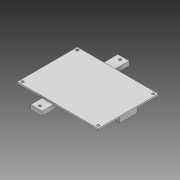
# Autodesk Inventor part: soporte_odroid_xu3
Saved by Autodesk Inventor 2018 (Build 220112000, 112)
## iProperties
Created: 2019-01-29
Part Number: soporte_odroid_xu3
Material: Genérico
Document SubType Name: Modeling
Designer: becar
Density: 1 g/cm^3
Appearance: Valor por defecto
Author: becar
Autodesk Inventor part; units mm, degrees
ref_plane "YZ Plane" through (0, 0, 0) normal (1, 0, 0) x (0, 1, 0)
ref_plane "XZ Plane" through (0, 0, 0) normal (0, 1, 0) x (-1, 0, 0)
ref_plane "XY Plane" through (0, 0, 0) normal (0, 0, 1) x (1, 0, 0)
sketch "Boceto1" plane through (0, 0, 0) normal (0, 0, 1) x (1, 0, 0)
  line L0 (0, 0) -> (87, 0)
  line L1 (87, 63) -> (0, 63)
  circle A0 centre (0, 63) radius 1.5
  circle A1 centre (87, 63) radius 1.5
  circle A2 centre (87, 0) radius 1.5
  circle A3 centre (0, 0) radius 1.5
  line L2 (0, -3) -> (87, -3)
  line L3 (87, -3) -> (90, -3)
  line L4 (90, -3) -> (90, 63)
  line L5 (90, 63) -> (90, 66)
  line L6 (90, 66) -> (0, 66)
  line L7 (0, 66) -> (-3, 66)
  line L8 (-3, 66) -> (-3, -3)
  line L9 (-3, -3) -> (0, -3)
  dimension "d0" = 87
  dimension "d1" = 63
  dimension "d2" = 3
  dimension "d3" = 3
  dimension "d4" = 3
  dimension "d5" = 3
  dimension "d8" = 3
  dimension "d9" = 3
  dimension "d10" = 3
  constraints: 20 end point, 4 centre point, 4 coincident, 4 point on line, 3 perpendicular, 2 horizontal, 1 collinear
  measures "d0" distance of L0.start L0.end
  measures "d1" distance of L0.end L1.start
  measures "d2" diameter of A0
  measures "d3" diameter of A1
  measures "d4" diameter of A2
  measures "d5" diameter of A3
  measures "d8" distance of L2.end L3.end
  measures "d9" distance of L4.end L5.end
  measures "d10" distance of L6.end L7.end
extrude "Extrusión1" add sketch "Boceto1" along normal blind 2
sketch "Boceto2" plane through (0, 0, 0) normal (0, 0, -1) x (-1, 0, 0)
  line L0 (0, 0) -> (0, -12)
  circle A0 centre (0, 63) radius 1.5 projected
  line L1 (0, 63) -> (0, 80)
  line L2 (0, 80) -> (-32, 80)
  line L3 (0, -12) -> (-32, -12)
  circle A1 centre (-32, 80) radius 1.5
  circle A2 centre (-32, -12) radius 1.5
  line L4 (-32, 80) -> (-25.5, 80)
  line L5 (-25.5, 80) -> (-25.5, 84)
  line L6 (-25.5, 84) -> (-38.5, 84)
  line L7 (-38.5, 84) -> (-38.5, 66)
  line L8 (-90, 66) -> (3, 66) projected
  line L9 (-25.5, 80) -> (-25.5, 66)
  line L10 (-38.5, -12) -> (-38.5, -2.9941)
  line L11 (-38.5, -12) -> (-38.5, -16)
  line L12 (-38.5, -16) -> (-25.5, -16)
  line L13 (-25.5, -16) -> (-25.5, -3)
  line L14 (3, -3) -> (-90, -3) projected
  line L15 (3, 66) -> (3, -3) projected
  line L16 (3, 31.5) -> (3, 41.5)
  line L17 (3, 31.5) -> (3, 21.5)
  line L18 (-90, -3) -> (-90, 66) projected
  line L19 (-90, 21.5) -> (-90, 41.5)
  line L20 (-90, 41.5) -> (-38.5, 41.5)
  line L21 (-38.5, 41.5) -> (-38.5, 66)
  line L22 (3, 41.5) -> (-25.5, 41.5)
  line L23 (-38.5, -2.9941) -> (-38.5, 21.5)
  line L24 (-25.5, 66) -> (-25.5, 41.5)
  line L25 (-25.5, -3) -> (-25.5, 21.5)
  line L26 (-38.5, 21.5) -> (-90, 21.5)
  line L27 (-25.5, 21.5) -> (3, 21.5)
  dimension "d13" = 12
  dimension "d14" = 17
  dimension "d15" = 32
  dimension "d16" = 3
  dimension "d17" = 3
  dimension "d18" = 6.5
  dimension "d19" = 4
  dimension "d20" = 13
  dimension "d21" = 4
  dimension "d22" = 10
  dimension "d23" = 10
  dimension "d24" = 20
  constraints: 48 end point, 11 point on line, 7 perpendicular, 4 vertical, 3 horizontal, 2 centre point, 2 coincident, 1 collinear, 1 midpoint
  measures "d13" distance of L0.start L0.end
  measures "d14" distance of L1.start L1.end
  measures "d15" distance of L1.end L2.end
  measures "d16" diameter of A1
  measures "d17" diameter of A2
  measures "d18" distance of L4.start L4.end
  measures "d19" distance of L4.end L5.end
  measures "d20" distance of L5.end L6.end
  measures "d21" distance of L10.start L11.end
  measures "d22" distance of L16.start L16.end
  measures "d23" distance of L16.start L17.end
  measures "d24" distance of L19.start L19.end
extrude "Extrusión2" add sketch "Boceto2" along normal blind 5 contours L13 L12 L11 L10 L14 | L14 L10 L23 L26 L18 L20 L21 L8 L24 L22 L15 L27 L25 | L8 L7 L6 L5 L9
sketch "Boceto3" plane through (0, 0, -5) normal (0, 0, -1) x (-1, 0, 0)
  circle A0 centre (-32, 80) radius 1.5 projected
  circle A1 centre (-32, 80) radius 3
  circle A2 centre (-32, -12) radius 1.5 projected
  circle A3 centre (-32, -12) radius 3
  point P0 (0, 0)
  dimension "d27" = 6
  dimension "d28" = 6
  constraints: 2 centre point, 2 coincident
  measures "d27" diameter of A1
  measures "d28" diameter of A3
extrude "Extrusión3" cut sketch "Boceto3" against normal blind 2
sketch "Boceto4" plane through (38.5, 41.5, 0) normal (0, 1, 0) x (1, 0, 0)
  line L0 (51.5, 0) -> (51.5, 5) projected
  line L1 (51.5, 0) -> (46.5, 0)
  line L2 (51.5, 0) -> (0, 0) projected
  line L3 (46.5, 0) -> (46.5, 2)
  line L4 (46.5, 2) -> (5, 2)
  line L5 (5, 2) -> (5, 0)
  line L6 (5, 0) -> (46.5, 0)
  line L7 (-41.5, 0) -> (-13, 0) projected
  line L8 (-13, 0) -> (-18, 0)
  line L9 (-18, 0) -> (-18, 2)
  line L10 (-18, 2) -> (-36.5, 2)
  line L11 (-36.5, 2) -> (-36.5, 0)
  line L12 (-36.5, 0) -> (-18, 0)
  point P0 (-38.5, 0)
  dimension "d31" = 5
  dimension "d32" = 2
  dimension "d33" = 41.5
  dimension "d34" = 5
  dimension "d35" = 18.5
  constraints: 20 end point, 7 perpendicular, 4 point on line, 1 collinear
  measures "d31" distance of L0.start L1.end
  measures "d32" distance of L1.end L3.end
  measures "d33" distance of L3.end L4.end
  measures "d34" distance of L7.end L8.end
  measures "d35" distance of L9.end L10.end
extrude "Extrusión4" cut sketch "Boceto4" against normal up to surface (20 mm away)
